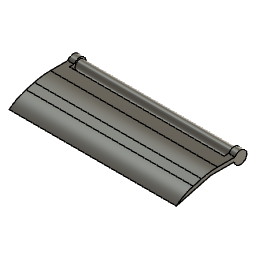
Hinge for micro switch cover v10 (Autodesk Fusion 360 design; units mm, degrees)
Autodesk Fusion 360 part; units mm, degrees
sketch "Sketch1" plane through (0, 0, 0) normal (1, 0, 0) x (0, 1, 0)
  line L0 (0, 0) -> (-0.5, 0)
  line L1 (-0.5, 0) -> (-0.5, -0.5)
  line L2 (-0.5, -0.5) -> (0, -0.5)
  line L3 (0, -0.5) -> (0, 0)
  constraint horizontal L0
  constraint vertical L1
  constraint horizontal L2
  constraint vertical L3
  constraint coincident L0.start L3.end
extrude "Extrude1" add sketch "Sketch1" along normal blind 1 makes body 1
sketch "Sketch2" plane through (1, 0, 0) normal (1, 0, 0) x (0, 1, 0)
  line L0 (0, -0.5) -> (0, 0)
  line L1 (0, 0) -> (-0.5, 0)
  line L2 (-0.5, 0) -> (-0.5, -0.5)
  line L3 (-0.5, -0.5) -> (0, -0.5)
  circle A0 centre (-0.25, -0.25) radius 1.5
  dimension "d3" = 3
  measures "d3" diameter of A0
extrude "Extrude2" add sketch "Sketch2" along normal blind 48 contours L0 L1 L2 L3 | A0 bodies 1
sketch "Sketch3" plane through (49, 0, 0) normal (1, 0, 0) x (0, 1, 0)
  circle A0 centre (-0.25, -0.25) radius 1.5
  line L0 (-1, 0.5) -> (0.5, 0.5)
  line L1 (0.5, 0.5) -> (0.5, -1)
  line L2 (0.5, -1) -> (-1, -1)
  line L3 (-1, -1) -> (-1, 0.5)
  constraint horizontal L0
  constraint vertical L1
  constraint horizontal L2
  constraint vertical L3
extrude "Extrude3" add sketch "Sketch3" along normal blind 1 separate body contours L0 L1 L2 L3 makes body 2
extrude "Extrude4" add 1 faces at (49, 0.7056, -0.5448) along direction (1, 0, 0) blind 1 on bodies 1 bodies 1 2
extrude "Extrude5" add 1 faces at (0.3333, -0.1667, 0) along direction (0, 0, 1) blind 0.5 on bodies 1 bodies 1
extrude "Extrude6" add 1 faces at (0.6667, -0.5, 0.1667) along direction (0, -1, 0) blind 0.5 on bodies 1 bodies 1
extrude "Extrude7" add 1 faces at (0.6667, -0.6667, -0.5) along direction (0, 0, -1) blind 0.5 on bodies 1 bodies 1
extrude "Extrude8" add 1 faces at (0.6667, 0, -0.5) along direction (0, 1, 0) blind 0.5 on bodies 1 bodies 1
sketch "Sketch5" plane through (50, 0, 0) normal (1, 0, 0) x (0, 1, 0)
  line L0 (-20, -7) -> (-18.2094, -7)
  line L1 (-20, -7) -> (-21.6158, -7)
  line L2 (-21.6158, -7) -> (-25.723, -7)
  line L3 (-25.723, -7) -> (-24.9973, -11.3371)
  line L4 (-24.9973, -11.3371) -> (-16.724, -10.4299)
  line L5 (-16.724, -10.4299) -> (-18.2094, -7)
  circle A0 centre (-0.25, -0.25) radius 1.5
  constraint horizontal L0
  constraint parallel L0 L1
  constraint parallel L1 L2
sketch "Sketch6" plane through (50, 0, 0) normal (1, 0, 0) x (0, 1, 0)
  circle A0 centre (-0.25, -0.25) radius 1.5
  circle A1 centre (-0.25, -0.25) radius 2
  dimension "d50" = 4
  constraint concentric A0 A1
  measures "d50" diameter of A1
extrude "Extrude21" add sketch "Sketch6" along normal blind 2 contours A0 | A1 bodies 1
extrude "Extrude22" cut 1 faces at (0, 0, -0.5) along direction (1, 0, 0) blind 1 on bodies 1 bodies 1
sketch "Sketch7" plane through (1, 0, 0) normal (-1, 0, 0) x (0, -1, 0)
  circle A0 centre (0.25, -0.25) radius 1.5
  circle A1 centre (0.25, -0.25) radius 2
  dimension "d55" = 4
  constraint concentric A0 A1
  measures "d55" diameter of A1
extrude "Extrude23" add sketch "Sketch7" along normal blind 2 contours A0 | A1 bodies 1
sketch "Sketch8" plane through (-1, 0, 0) normal (-1, 0, 0) x (0, -1, 0)
  circle A0 centre (0.25, -0.25) radius 2
  line L0 (2.0007, 0.717) -> (10.1126, 0.717)
  line L1 (10.1126, 0.717) -> (20.9443, -2.2031)
  line L2 (20.9443, -2.2031) -> (20.6162, -3.4203)
  line L3 (20.6162, -3.4203) -> (9.689, -0.4744)
  line L4 (9.689, -0.4744) -> (2.2325, -0.5138)
  constraint coincident A0 L0.start
  constraint horizontal L0
  constraint perpendicular L1 L2
  constraint perpendicular L2 L3
  constraint coincident A0 L4.end
extrude "Extrude24" add sketch "Sketch8" against normal blind 53 contours A0 L0 L1 L2 L3 L4 bodies 1
sketch "Sketch9" plane through (0, 0, 0.717) normal (0, 0, 1) x (-1, 0, 0)
  line L0 (1, 2.0007) -> (1, 10.1126)
  line L1 (1, 10.1126) -> (-52, 10.1126)
  line L2 (-52, 10.1126) -> (-52, 2.0007)
  line L3 (-50, 2.0007) -> (-1, 2.0007)
  line L4 (-1, 2.0007) -> (1, 2.0007)
  line L5 (-1, 2.0007) -> (-50, 2.0007)
  line L6 (-50, 2.0007) -> (-50, 3.4554)
  line L7 (-50, 3.4554) -> (-1, 3.4554)
  line L8 (-1, 3.4554) -> (-1, 2.0007)
  line L9 (-52, 2.0007) -> (-50, 2.0007)
  constraint horizontal L5
  constraint vertical L6
  constraint horizontal L7
  constraint vertical L8
  constraint coincident L3.end L4.start
extrude "Extrude25" cut sketch "Sketch9" against normal blind 10 contours L3 L5 L6 L7 L8 bodies 1
fillet "Fillet5" radius 14.5 1 edges at (25.5, -20.9443, -2.2031) on bodies 1
fillet "Fillet6" radius 19.5 1 edges at (25.5, -10.1126, 0.717) on bodies 1
